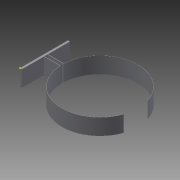
# Autodesk Inventor part: Part151
Saved by Autodesk Inventor 2015 (Build 190159000, 159)
## iProperties
Created: 2015-01-10
Part Number: Part151
Material: Generic
Document SubType Name: Modeling
Designer: bergjos18
Density: 1 g/cm^3
Appearance: Default
Author: bergjos18
Autodesk Inventor part; units mm, degrees
ref_plane "YZ Plane" through (0, 0, 0) normal (1, 0, 0) x (0, 1, 0)
ref_plane "XZ Plane" through (0, 0, 0) normal (0, 1, 0) x (-1, 0, 0)
ref_plane "XY Plane" through (0, 0, 0) normal (0, 0, 1) x (1, 0, 0)
sketch "Sketch1" plane through (0, 0, 0) normal (1, 0, 0) x (0, 1, 0)
  point P0 (0, 0)
sketch "Sketch2" plane through (0, 0, 0) normal (1, 0, 0) x (0, 1, 0)
  line L0 (0, 0) -> (-101.6, 0)
  line L1 (-101.6, 0) -> (-101.6, -304.8)
  line L2 (-101.6, -304.8) -> (0, -304.8)
  line L3 (0, -304.8) -> (0, 0)
  dimension "d0" = 101.6
  dimension "d1" = 304.8
  constraints: 8 end point, 2 parallel, 1 coincident, 1 horizontal, 1 perpendicular
  measures "d0" distance of L2.end L1.end
  measures "d1" distance of L1.end L0.end
extrude "Extrusion1" add sketch "Sketch2" along normal blind 12.7
sketch "Sketch3" plane through (0, 0, 0) normal (0, 1, 0) x (1, 0, 0)
  line L0 (12.7, 304.8) -> (12.7, 0) projected
  line L1 (12.7, 0) -> (12.7, 304.8) projected
  line L2 (12.7, 139.7) -> (114.3, 139.7)
  line L3 (114.3, 139.7) -> (114.3, 142.24)
  line L4 (114.3, 142.24) -> (12.7, 142.24)
  line L5 (12.7, 142.24) -> (12.7, 139.7)
  line L6 (12.7, 162.56) -> (114.3, 162.56)
  line L7 (114.3, 162.56) -> (114.3, 165.1)
  line L8 (114.3, 165.1) -> (12.7, 165.1)
  line L9 (12.7, 165.1) -> (12.7, 162.56)
  line L10 (0, 304.8) -> (12.7, 304.8) projected
  circle A0 centre (355.6, 152.4) radius 241.3
  circle A1 centre (355.6, 152.4) radius 240.03
  point P0 (0, 0)
  dimension "d6" = 2.54
  dimension "d7" = 2.54
  dimension "d8" = 139.7
  dimension "d9" = 139.7
  dimension "d10" = 482.6
  dimension "d11" = 342.9
  dimension "d12" = 101.6
  dimension "d13" = 480.06
  constraints: 16 end point, 4 parallel, 3 point on line, 2 centre point, 2 horizontal, 2 perpendicular, 1 coincident
  measures "d6" distance of L8.end L6.start
  measures "d7" distance of L4.end L2.start
  measures "d8" distance of L2.start L0.end
  measures "d9" distance from line of L10 L8.end
  measures "d10" diameter of A0
  measures "d11" distance from line of A0.centre L0
  measures "d12" distance of L7.end L8.end
  measures "d13" diameter of A1
extrude "Extrusion2" add sketch "Sketch3" against normal blind 101.6
sketch "Sketch4" plane through (355.6, 0, -152.4) normal (0, 1, 0) x (1, 0, 0)
  circle A0 centre (0, 0) radius 241.3 projected
  arc A1 (-241.0857, 10.1682) -> (-241.0043, -10.1422) centre (-39.0277, 0.8227) ccw
  circle A2 centre (0, 0) radius 240.03 projected
  arc A3 (-239.8145, 10.1682) -> (-239.8156, -10.1422) centre (0, 0) ccw
  line L0 (-241.0043, -10.1422) -> (-239.8156, -10.1422)
  line L1 (-241.0857, 10.1682) -> (-239.8145, 10.1682)
  point P0 (-355.6, -152.4)
  constraints: 6 point on circle, 4 end point, 2 centre point, 1 horizontal, 1 parallel, 2 other
extrude "Extrusion3" cut sketch "Sketch4" against normal blind 101.6 contours L1 A2 L0 A1 A0 | A0 A1 picked at (-240.3417, 6.7814)
sketch "Sketch5" plane through (0, 0, 0) normal (0, 1, 0) x (1, 0, 0)
  arc A0 (115.7844, 142.2578) -> (115.7855, 162.5682) centre (355.6, 152.4) ccw projected
  arc A1 (582.8083, 74.9997) -> (583.5551, 227.5722) centre (355.6, 152.4) ccw
  arc A2 (114.3, 152.4) -> (114.5143, 162.5682) centre (355.6, 152.4) ccw projected
  arc A3 (584.1495, 74.9997) -> (584.892, 227.5722) centre (355.6, 152.4) ccw
  line L0 (582.8083, 74.9997) -> (584.1495, 74.9997)
  line L1 (584.892, 227.5722) -> (583.5551, 227.5722)
  point P0 (0, 0)
  constraints: 8 point on circle, 4 end point, 2 centre point, 1 horizontal, 1 parallel
extrude "Extrusion4" cut sketch "Sketch5" against normal blind 101.6
body "Solid1"
